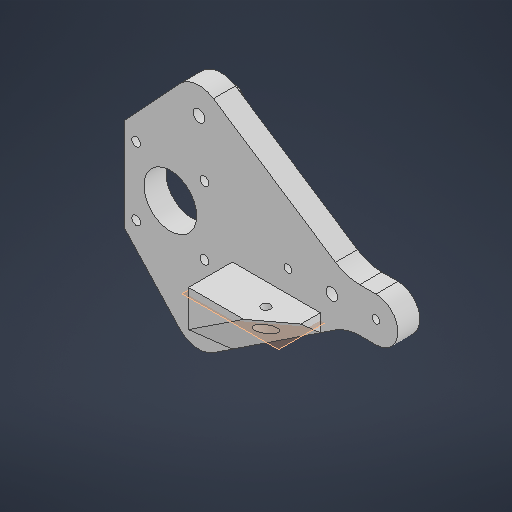
# Autodesk Inventor part: y axis motor holder
Saved by Autodesk Inventor 2025.1 (Build 291241000, 241)
## iProperties
Created: 2025-02-02
Part Number: y axis motor holder
Material: Generic
Document SubType Name: Modeling
Designer: jerem
Density: 1 g/cm^3
Appearance: Default
Author: jerem
Autodesk Inventor part; units mm, degrees
ref_plane "YZ Plane" through (0, 0, 0) normal (1, 0, 0) x (0, 1, 0)
ref_plane "XZ Plane" through (0, 0, 0) normal (0, 1, 0) x (-1, 0, 0)
ref_plane "XY Plane" through (0, 0, 0) normal (0, 0, 1) x (1, 0, 0)
sketch "Sketch1" plane through (0, 0, 0) normal (0, 0, 1) x (1, 0, 0)
  line L0 (0, 0) -> (30.25, 0) construction
  line L1 (0, 0) -> (-30.25, 0) construction
  line L2 (-30.25, 0) -> (-30.25, 40) construction
  line L3 (-30.25, 0) -> (-30.25, -40) construction
  circle A0 centre (-30.25, 40) radius 2.7
  circle A1 centre (-30.25, -40) radius 2.7
  circle A2 centre (30.25, 0) radius 2.7
  circle A3 centre (-30.25, 40) radius 12
  circle A4 centre (-30.25, -40) radius 12
  circle A5 centre (30.25, 0) radius 12
  line L4 (36.8682, -10.01) -> (-23.6318, -50.01)
  line L5 (-42.25, 40) -> (-42.25, -40)
  line L6 (-23.6318, 50.01) -> (36.8682, 10.01)
  line L7 (30.25, 0) -> (50.25, 0) construction
  circle A6 centre (50.25, 0) radius 10
  circle A7 centre (50.25, 0) radius 1.75
  line L8 (50.2575, 10) -> (36.8682, 10.01)
  line L9 (50.2575, -10) -> (36.8682, -10.01)
  line L10 (-27.75, -15.5) -> (-58.75, -15.5) construction
  line L11 (-58.75, -15.5) -> (-58.75, 15.5) construction
  line L12 (-58.75, 15.5) -> (-27.75, 15.5) construction
  line L13 (-27.75, 15.5) -> (-27.75, -15.5) construction
  line L14 (-27.75, -15.5) -> (-58.75, 15.5) construction
  line L15 (-58.75, -15.5) -> (-27.75, 15.5) construction
  line L16 (-22.25, -21) -> (-64.25, -21) construction
  line L17 (-64.25, -21) -> (-64.25, 21)
  line L18 (-64.25, 21) -> (-22.25, 21) construction
  line L19 (-22.25, 21) -> (-22.25, -21) construction
  line L20 (-22.25, -21) -> (-64.25, 21) construction
  line L21 (-64.25, -21) -> (-22.25, 21) construction
  line L22 (-43.25, 0) -> (-42.25, 0) construction
  circle A8 centre (-27.75, 15.5) radius 2
  circle A9 centre (-58.75, 15.5) radius 2
  circle A10 centre (-58.75, -15.5) radius 2
  circle A11 centre (-27.75, -15.5) radius 2
  line L23 (-64.25, 21) -> (-39.0465, 48.1622)
  line L24 (-64.25, -21) -> (-39.0465, -48.1622)
  circle A12 centre (-43.25, 0) radius 12
  circle A13 centre (10.25, 0) radius 1.75
  point P0 (41.35, -4.5596)
  point P1 (41.35, 4.5596)
  dimension "d0" = 60.5
  dimension "d1" = 5.4
  dimension "d2" = 80
  dimension "d3" = 24
  dimension "d57" = 20
  dimension "d58" = 20
  dimension "d61" = 31
  dimension "d63" = 42
  dimension "d65" = 1
  dimension "d66" = 4
  dimension "d67" = 4
  dimension "d68" = 4
  dimension "d69" = 4
  dimension "d70" = 3.5
  dimension "d71" = 24
  dimension "d74" = 3.5
  dimension "d75" = 20
  constraints: 50 end point, 14 centre point, 13 coincident, 10 point on circle, 9 tangent, 6 horizontal, 5 midpoint, 4 equal length, 4 equal radius, 4 parallel, 3 perpendicular, 2 vertical, 1 point on line
  measures "d0" distance of L0.end L1.end
  measures "d1" diameter of A0
  measures "d2" distance of L3.end L2.end
  measures "d3" diameter of A3
  measures "d57" distance of L7.start L7.end
  measures "d58" diameter of A6
  measures "d61" distance of L10.end L11.end
  measures "d63" distance of L16.end L17.end
  measures "d65" distance of L22.end L22.start
  measures "d66" diameter of A8
  measures "d67" diameter of A9
  measures "d68" diameter of A10
  measures "d69" diameter of A11
  measures "d70" diameter of A7
  measures "d71" diameter of A12
  measures "d74" diameter of A13
  measures "d75" distance of L0.end A13.centre
extrude "Extrusion1" add sketch "Sketch1" against normal blind 10 contours A3 | A3 L6 A5 L4 A4 L5 A12 | L5 A12 A4 L24 L17 L23 A3 | A5 A6 | L8 A6 A5 | A5 A6 L9 | A6 A5 | A5 A6 | A4
sketch "Sketch4" plane through (0, 0, -10) normal (0, 0, -1) x (1, 0, 0)
  circle A0 centre (-30.25, -40) radius 4
  circle A1 centre (30.25, 0) radius 4
  circle A2 centre (-30.25, 40) radius 4
  arc A3 (-23.6318, 50.01) -> (-39.0465, 48.1622) centre (-30.25, 40) ccw projected
  arc A4 (-39.0465, -48.1622) -> (-23.6318, -50.01) centre (-30.25, -40) ccw projected
  line L0 (-23.6318, -50.01) -> (36.8682, -10.01) projected
  line L1 (36.8682, -10.01) -> (50.2575, -10) projected
  arc A5 (50.2575, -10) -> (50.2575, 10) centre (50.25, 0) ccw projected
  line L2 (50.2575, 10) -> (36.8682, 10.01) projected
  line L3 (36.8682, 10.01) -> (-23.6318, 50.01) projected
  circle A6 centre (-30.25, 40) radius 2.7 projected
  circle A7 centre (30.25, 0) radius 2.7 projected
  circle A8 centre (-30.25, -40) radius 2.7 projected
  circle A9 centre (50.25, 0) radius 1.75 projected
  line L4 (-39.0465, 48.1622) -> (-64.25, 21) projected
  line L5 (-64.25, 21) -> (-64.25, -21) projected
  line L6 (-64.25, -21) -> (-39.0465, -48.1622) projected
  point P0 (0, 0)
  dimension "d26" = 8
  constraints: 3 centre point, 2 equal radius, 1 coincident
  measures "d26" diameter of A0
extrude "Extrusion4" add sketch "Sketch4" along normal blind 6.45 contours A0 | A1 | A2
chamfer "Chamfer2" distance 6 angle 45 3 edges at (26.25, 0, -10) (-34.25, -40, -10) (-34.25, 40, -10)
fillet "Fillet1" radius 20 2 edges at (36.8682, 10.01, -5) (36.8682, -10.01, -5)
sketch "Sketch5" plane through (0, 0, 0) normal (0, 0, 1) x (1, 0, 0)
  line L0 (0, 0) -> (0, -10) construction
  line L1 (0, -10) -> (-15, -10)
  line L2 (0, -10) -> (25, -10)
  line L3 (42.8738, -10.0055) -> (50.2575, -10) projected
  arc A0 (50.2575, -10) -> (50.2575, 10) centre (50.25, 0) ccw projected
  line L4 (50.2575, 10) -> (42.8738, 10.0055) projected
  arc A1 (31.8585, 13.3222) -> (42.8738, 10.0055) centre (42.8887, 30.0055) ccw projected
  line L5 (31.8585, 13.3222) -> (-23.6318, 50.01) projected
  arc A2 (-23.6318, 50.01) -> (-39.0465, 48.1622) centre (-30.25, 40) ccw projected
  line L6 (-39.0465, 48.1622) -> (-64.25, 21) projected
  line L7 (-64.25, 21) -> (-64.25, -21) projected
  line L8 (-64.25, -21) -> (-39.0465, -48.1622) projected
  arc A3 (-39.0465, -48.1622) -> (-23.6318, -50.01) centre (-30.25, -40) ccw projected
  line L9 (-23.6318, -50.01) -> (31.8585, -13.3222) projected
  arc A4 (42.8738, -10.0055) -> (31.8585, -13.3222) centre (42.8887, -30.0055) ccw projected
  circle A5 centre (30.25, 0) radius 2.7 projected
  circle A6 centre (50.25, 0) radius 1.75 projected
  circle A7 centre (-30.25, -40) radius 2.7 projected
  circle A8 centre (-27.75, -15.5) radius 2 projected
  circle A9 centre (-27.75, 15.5) radius 2 projected
  circle A10 centre (-58.75, 15.5) radius 2 projected
  circle A11 centre (-58.75, -15.5) radius 2 projected
  circle A12 centre (-43.25, 0) radius 12 projected
  circle A13 centre (-30.25, 40) radius 2.7 projected
  line L10 (-15, -10) -> (-15, -44.303)
  line L11 (25, -10) -> (25, -17.8567)
  dimension "d72" = 10
  dimension "d73" = 15
  dimension "d76" = 25
  constraints: 10 end point, 2 point on line, 2 vertical, 1 horizontal, 1 parallel, 1 perpendicular
  measures "d72" distance of L0.start L0.end
  measures "d73" distance of L0.end L1.end
  measures "d76" distance of L0.end L2.end
extrude "Extrusion6" add sketch "Sketch5" along normal blind 20 contours L2 L11 L9 L10 L1
sketch "Sketch6" plane through (-15, -10, 0) normal (0, 1, 0) x (1, 0, 0)
  line L0 (27, 0) -> (23.5, 0) projected
  line L1 (25.25, 0) -> (25.25, -10) construction
  circle A0 centre (25.25, -10) radius 2
  point P0 (15, 0)
  dimension "d82" = 10
  dimension "d83" = 4
  constraints: 2 end point, 1 centre point, 1 coincident, 1 midpoint, 1 perpendicular
  measures "d82" distance of L1.start L1.end
  measures "d83" diameter of A0
extrude "Extrusion7" cut sketch "Sketch6" against normal through all
ref_plane "Work Plane2" through (-15, -13, 0) normal (0, 1, 0) x (1, 0, 0)
sketch "Sketch7" plane through (-15, -13, 0) normal (0, 1, 0) x (1, 0, 0)
  circle A0 centre (25.25, -10) radius 2 projected
  circle A1 centre (25.25, -10) radius 4.5
  point P0 (15, 0)
  dimension "d87" = 9
  constraints: 1 centre point, 1 coincident
  measures "d87" diameter of A1
extrude "Extrusion8" cut sketch "Sketch7" against normal through all
chamfer "Chamfer6" distance 14.75 distance2 20 1 edges at (5, -31.0799, 20) measured on face at (4.7242, -30.6628, 20)
equation "\"b\" = 2"
body "Solid1"
